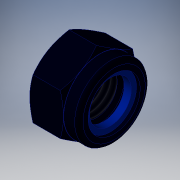
# Autodesk Inventor part: BN 161 1118811 prevailing torque type hex lock nut M20
Saved by Autodesk Inventor 2019 (Build 230136000, 136)
## iProperties
Created: 2023-02-02
Part Number: BN 161 1118811 prevailing torque type hex lock nut M20
Material: Generic
Catalog Web Link: www.cadenas.de
Description: BN 161-Prevailing torque type hex lock nuts thin type, with polyamide insert (DIN 985), cl. 6, zinc plated blue
Vendor: BOSSARD
Document SubType Name: Modeling
Designer: psAdmin
Manufacturer: BOSSARD
Mass: 9.6861 g
Surface Area: 42.4229 cm^2
Volume: 9.6861 cm^3
Density: 1 g/cm^3
Appearance: PSOLRGB-10-17-107
Category: PARTsolutions
Company: BOSSARD
Title: BN 161 1118811 prevailing torque type hex lock nut M20
Author: Cadenas PARTsolutions
Comments: Prevailing torque type hex lock nuts thin type, with polyamide insert (DIN 985), cl. 6, zinc plated blue
PSOL_IDENT_0: {$CADENAS_DATA/23d-libs/bossard/bossard_new/01/01_300/01_300_600/01_300_600_30/bn_161_20227_80035/bn
PSOL_IDENT_1: _161.prj},265 {M=Nenngewinde},{VTYP=3D},{NB=BN 161 1118811 prevailing torque type hex lock nut M20},
PSOL_IDENT_2: {LINA=BN 161 1118811 prevailing torque type hex lock nut M20},{NN=BN 161},{DATE=09.05.2022 06:08:19}
PSOL_IDENT_3: ,{GEOMDATE=21.09.2021 13:24:40},{VERSION=},{LINEID=210},{WBVAR=},{WBNUMERIC=}  {NB=BN 161 1118811 pr
PSOL_IDENT_4: evailing torque type hex lock nut M20},{LINA=BN 161 1118811 prevailing torque type hex lock nut M20}
PSOL_IDENT_5: ,{KT=X},{NENN=M20},{CNSORDERNO=1118811},{BNARTNR=1118811},{BNNORM1=DIN 985},{BNMAT=Stahl 6},{CNSMAT=
PSOL_IDENT_6: Stahl 6},{BNSURFACE=verzinkt-blau},{D=20.000},{D1=17.294},{P=2.500},{DIN962THREAD=},{XLH=0},{DIN962O
PSOL_IDENT_7: PT2=},{DA=21.600},{M=20.000},{M1=14.000},{S=30.000},{SKD2=3.000},{OPTIONS2L='',' - ','din_962_std.jp
PSOL_IDENT_8: g','-SK','SK Drahtloch','din_962_s_4.jpg'},{VERS=1.000},{DIN962FTHREAD=0}
NB: BN 161 1118811 prevailing torque type hex lock nut M20
NN: BN 161
NT: Prevailing torque type hex lock nuts thin type, with polyamide insert (DIN 985), cl. 6, zinc plated blue
NBSYN: BN 161 $BNARTNR. prevailing torque type hex lock nut $NENN.
LINA: BN 161 1118811 prevailing torque type hex lock nut M20
CATALOG: Bossard Catalog
ROWDESC: M20
OFFICIAL_STANDARD_NUMBERS: DIN 985
BNARTNR: 1118811
BNNORM1: DIN 985
BNMAT: Steel 6
BNSURFACE: zinc plated blue
D: 20
D1: 17.294
P: 2.5
DA: 21.6
M: 20
M1: 14
S: 30
SUPPLIER: BOSSARD
ARTICLENO: BN 161 1118811 prevailing torque type hex lock nut M20
BOMINFO: BN 161 1118811 prevailing torque type hex lock nut M20
CREATOR: CADENAS GmbH
Autodesk Inventor part; units mm, degrees
sketch "Sketch_1" plane through (0, 0, 0) normal (0, 0, 1) x (1, 0, 0)
  line L0 (20, 0) -> (0, 0)
  line L1 (0, 0) -> (0, 18)
  line L2 (0, 18) -> (20, 18)
  line L3 (20, 18) -> (20, 10.8)
  line L4 (20, 10.8) -> (18.5, 10.8)
  line L5 (18.5, 10.8) -> (18.5, 8.647)
  line L6 (18.5, 8.647) -> (15.5, 8.647)
  line L7 (15.5, 8.647) -> (15.5, 10.8)
  line L8 (15.5, 10.8) -> (14, 10.8)
  line L9 (14, 10.8) -> (14, 0)
  line L10 (14, 0) -> (0, 0)
  constraints: 22 end point
revolve "Revolution1" add sketch "Sketch_1" angle 360 about axis through (20, 0, 0) along (-1, 0, 0)
sketch "Sketch_2" plane through (0, 0, 0) normal (1, 0, 0) x (0, 1, 0)
  line L0 (30, 30) -> (-30, 30)
  line L1 (-30, 30) -> (-30, -30)
  line L2 (-30, -30) -> (30, -30)
  line L3 (30, -30) -> (30, 30)
  line L4 (-8.6603, 15) -> (-17.3205, 0)
  line L5 (-17.3205, 0) -> (-8.6603, -15)
  line L6 (-8.6603, -15) -> (8.6603, -15)
  line L7 (8.6603, -15) -> (17.3205, 0)
  line L8 (17.3205, 0) -> (8.6603, 15)
  line L9 (8.6603, 15) -> (-8.6603, 15)
  constraints: 20 end point
extrude "Extrusion1" cut sketch "Sketch_2" along normal mid plane 42
sketch "Sketch_8" plane through (0, 0, 0) normal (0, 0, 1) x (1, 0, 0)
  line L0 (20, 0) -> (0, 0)
  line L1 (14, 18) -> (14, 14.9)
  line L2 (14, 14.9) -> (20, 14.9)
  line L3 (20, 14.9) -> (20, 18)
  line L4 (20, 18) -> (14, 18)
  constraints: 10 end point
revolve "Revolution2" cut sketch "Sketch_8" angle 360 about axis through (20, 0, 0) along (1, 0, 0)
sketch "Sketch_4" plane through (0, 0, 0) normal (0, 0, 1) x (1, 0, 0)
  line L0 (14, 0) -> (0, 0)
  line L1 (0, 0) -> (0, 10.8)
  line L2 (0, 10.8) -> (2.153, 8.647)
  line L3 (2.153, 8.647) -> (12.647, 8.647)
  line L4 (12.647, 8.647) -> (14, 10)
  line L5 (14, 10) -> (14, 0)
  line L6 (14, 0) -> (0, 0)
  constraints: 14 end point
revolve "Revolution3" cut sketch "Sketch_4" angle 360 about axis through (14, 0, 0) along (1, 0, 0)
thread "Thread1" size "M20x2.5" class "6H" standard "ISO Metric profile" full length
sketch "Sketch_5" plane through (0, 0, 0) normal (0, 0, 1) x (1, 0, 0)
  line L0 (20, 0) -> (0, 0)
  line L1 (17.8, 15) -> (17.9, 15)
  arc A0 (20, 12.9) -> (17.9, 15) centre (17.9, 12.9) ccw
  line L2 (20, 12.9) -> (20.1, 12.9)
  line L3 (20.1, 12.9) -> (20.1, 22.5)
  line L4 (20.1, 22.5) -> (17.8, 22.5)
  line L5 (17.8, 22.5) -> (17.8, 15)
  constraints: 12 end point, 2 point on circle, 1 centre point
revolve "Revolution4" cut sketch "Sketch_5" angle 360 about axis through (20, 0, 0) along (1, 0, 0)
sketch "Sketch_6" plane through (0, 0, 0) normal (0, 0, 1) x (1, 0, 0)
  line L0 (20, 0) -> (0, 0)
  line L1 (-1, 15) -> (0, 15)
  line L2 (0, 15) -> (4.3301, 22.5)
  line L3 (4.3301, 22.5) -> (9.6699, 22.5)
  line L4 (9.6699, 22.5) -> (14, 15)
  line L5 (14, 15) -> (15.5, 15)
  line L6 (15.5, 15) -> (15.5, 25.5)
  line L7 (15.5, 25.5) -> (-1, 25.5)
  line L8 (-1, 25.5) -> (-1, 15)
  constraints: 18 end point
revolve "Revolution5" cut sketch "Sketch_6" angle 360 about axis through (20, 0, 0) along (1, 0, 0)
ref_plane "IP1_XY" through (0, 0, 0) normal (1, 0, 0) x (0, 0, -1)
ref_plane "IP1_YZ" through (0, 0, 0) normal (0, 0, -1) x (0, 1, 0)
ref_plane "IP1_ZX" through (0, 0, 0) normal (0, 1, 0) x (1, 0, 0)
ref_plane "IP2_XY" through (20, 0, 0) normal (1, 0, 0) x (0, 0, -1)
ref_plane "IP2_YZ" through (20, 0, 0) normal (0, 0, -1) x (0, 1, 0)
ref_plane "IP2_ZX" through (20, 0, 0) normal (0, 1, 0) x (1, 0, 0)
body "Solid1"
